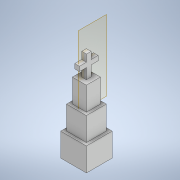
# Autodesk Inventor part: tiered-king
Saved by Autodesk Inventor 2021 (Build 250183000, 183)
## iProperties
Created: 2021-01-20
Part Number: tiered-king
Material: Generic
Document SubType Name: Modeling
Designer: Luke Kamols
Density: 1 g/cm^3
Appearance: Default
Author: Luke Kamols
Autodesk Inventor part; units mm, degrees
ref_plane "YZ Plane" through (0, 0, 0) normal (1, 0, 0) x (0, 1, 0)
ref_plane "XZ Plane" through (0, 0, 0) normal (0, 1, 0) x (-1, 0, 0)
ref_plane "XY Plane" through (0, 0, 0) normal (0, 0, 1) x (1, 0, 0)
sketch "Sketch1" plane through (0, 0, 0) normal (0, 1, 0) x (-1, 0, 0)
  line L0 (0, 0) -> (12, 0)
  line L1 (12, 0) -> (12, -12)
  line L2 (12, -12) -> (0, -12)
  line L3 (0, -12) -> (0, 0)
  dimension "d0" = 12
  dimension "d1" = 12
  constraints: 8 end point, 2 parallel, 1 horizontal, 1 perpendicular
  measures "d0" distance of L1.end L2.end
  measures "d1" distance of L0.end L1.end
extrude "Extrusion1" add sketch "Sketch1" along normal blind 20
ref_plane "Work Plane1" through (-6, 0, 0) normal (1, 0, 0) x (0, 0, -1)
sketch "Sketch2" plane through (-6, 0, 0) normal (1, 0, 0) x (0, 0, -1)
  line L0 (0, 20) -> (12, 20) projected
  line L1 (6, 20) -> (4, 20)
  line L2 (12, 20) -> (0, 20) projected
  line L3 (4, 20) -> (4, 29)
  line L4 (4, 29) -> (-2, 29)
  line L5 (-2, 29) -> (-2, 33)
  line L6 (-2, 33) -> (4, 33)
  line L7 (4, 33) -> (4, 39)
  line L8 (4, 39) -> (8, 39)
  line L9 (8, 39) -> (8, 33)
  line L10 (8, 33) -> (14, 33)
  line L11 (14, 33) -> (14, 29)
  line L12 (14, 29) -> (3, 29)
  line L13 (3, 29) -> (3, 20)
  line L14 (8, 29) -> (8, 20)
  line L15 (6, 20) -> (8, 20)
  point P0 (0, 0)
  dimension "d4" = 2
  dimension "d5" = 9
  dimension "d6" = 6
  dimension "d7" = 4
  dimension "d8" = 6
  dimension "d9" = 4
  dimension "d10" = 6
  constraints: 28 end point, 9 perpendicular, 6 point on line, 1 collinear, 1 horizontal, 1 midpoint, 1 vertical
  measures "d4" distance of L1.start L1.end
  measures "d5" distance of L1.end L3.end
  measures "d6" distance of L3.end L4.end
  measures "d7" distance of L4.end L5.end
  measures "d8" distance of L6.end L7.end
  measures "d9" distance of L7.end L8.end
  measures "d10" distance of L9.end L10.end
extrude "Extrusion2" add sketch "Sketch2" along normal mid plane 4 contours L3 L12 L14 L0 | L4 L5 L6 L7 L8 L9 L10 L11 L12
sketch "Sketch3" plane through (0, 0, 0) normal (0, -1, 0) x (1, 0, 0)
  line L0 (-12, 0) -> (0, 0) projected
  line L1 (0, 0) -> (0, -12) projected
  line L2 (0, 0) -> (2.5, 0)
  line L3 (2.5, 0) -> (2.5, 2.5)
  line L4 (2.5, 2.5) -> (-14.5, 2.5)
  line L5 (-14.5, 2.5) -> (-14.5, -14.5)
  line L6 (-14.5, -14.5) -> (2.5, -14.5)
  line L7 (2.5, -14.5) -> (2.5, 2.5)
  dimension "d15" = 2.5
  dimension "d16" = 2.5
  dimension "d17" = 17
  dimension "d18" = 17
  constraints: 12 end point, 2 horizontal, 2 parallel, 2 perpendicular
  measures "d15" distance of L0.end L2.end
  measures "d16" distance of L2.end L3.end
  measures "d17" distance of L6.end L5.end
  measures "d18" distance of L5.end L4.end
extrude "Extrusion3" add sketch "Sketch3" along normal blind 20
sketch "Sketch4" plane through (0, -20, 0) normal (0, -1, 0) x (1, 0, 0)
  line L0 (2.5, -14.5) -> (2.5, 2.5) projected
  line L1 (2.5, 2.5) -> (2.5, 5)
  line L2 (2.5, 5) -> (5, 5)
  line L3 (5, 5) -> (-17, 5)
  line L4 (-17, 5) -> (-17, -17)
  line L5 (-17, -17) -> (5, -17)
  line L6 (5, -17) -> (5, 5)
  point P0 (0, 0)
  dimension "d21" = 2.5
  dimension "d22" = 2.5
  dimension "d23" = 22
  dimension "d24" = 22
  constraints: 12 end point, 2 parallel, 2 perpendicular, 1 horizontal, 1 vertical
  measures "d21" distance of L0.end L1.end
  measures "d22" distance of L1.end L2.end
  measures "d23" distance of L5.end L4.end
  measures "d24" distance of L4.end L3.end
extrude "Extrusion4" add sketch "Sketch4" along normal blind 20
body "Solid1"
